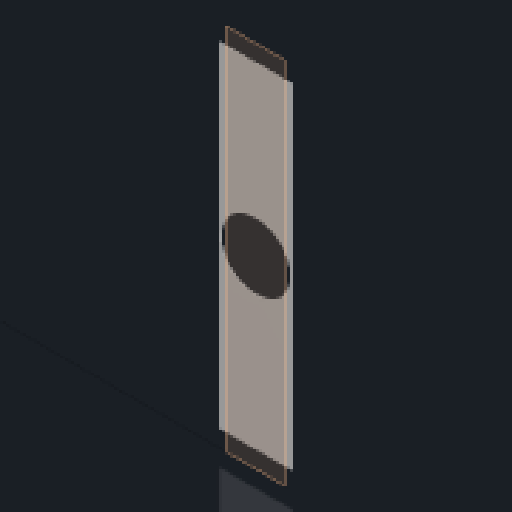
# Autodesk Inventor part: CARCASA_ALUM_2
Saved by Autodesk Inventor 2024.3 (Build 283343000, 343)
## iProperties
Created: 2024-05-15
Part Number: CARCASA_ALUM_2
Material: Generic
Document SubType Name: Sheet Metal
Designer: Niler
Density: 1 g/cm^3
Sheet Metal Rule: Default_mm
Appearance: Default
Author: Niler
Autodesk Inventor part; units mm, degrees
ref_plane "YZ Plane" through (0, 0, 0) normal (1, 0, 0) x (0, 1, 0)
ref_plane "XZ Plane" through (0, 0, 0) normal (0, 1, 0) x (-1, 0, 0)
ref_plane "XY Plane" through (0, 0, 0) normal (0, 0, 1) x (1, 0, 0)
ref_plane "Work Plane1" through (0, 0, 0) normal (0, 0, 1) x (1, 0, 0)
sketch "Sketch1" plane through (0, 0, 0) normal (0, 0, 1) x (1, 0, 0)
  line L0 (-90.0071, -785) -> (-90.0071, 235)
  line L1 (134.6291, -785) -> (-90.0071, -785)
  line L2 (134.6291, -785) -> (134.6291, 235)
  line L3 (-90.0071, 235) -> (134.6291, 235)
  spline S0 degree 3 poles (-83.4665, -275) (-83.4665, -270.5526) (-82.9168, -262.7698) (-81.2022, -254.0249) (-79.4626, -247.5768) (-78.0785, -243.3409) (-76.0752, -238.1427) (-74.2575, -234.0687) (-71.7257, -229.0988) (-69.4967, -225.2274) (-66.4671, -220.5344) (-63.8533, -216.9028) (-60.3609, -212.5309) (-57.3922, -209.1725) (-53.4761, -205.1609) (-50.1847, -202.1053) (-45.8867, -198.4886) (-42.3073, -195.7614) (-37.6715, -192.5693) (-33.84, -190.1925) (-28.9123, -187.4503) (-24.8659, -185.4423) (-19.6933, -183.1709) (-15.4701, -181.5469) (-10.1006, -179.7632) (-5.7393, -178.5349) (-0.2217, -177.2517) (4.2386, -176.428) (9.8552, -175.6545) (14.375, -175.2412) (20.0412, -174.9828) (24.5808, -174.9828) (30.247, -175.2412) (34.7668, -175.6545) (40.3834, -176.428) (44.8437, -177.2517) (50.3613, -178.5349) (54.7226, -179.7632) (60.092, -181.5469) (64.3153, -183.1709) (69.4878, -185.4423) (73.5343, -187.4503) (78.4619, -190.1925) (82.2935, -192.5693) (86.9292, -195.7614) (90.5087, -198.4886) (94.8067, -202.1053) (98.098, -205.1609) (102.0141, -209.1725) (104.9829, -212.5309) (108.4753, -216.9028) (111.089, -220.5344) (114.1187, -225.2274) (116.3477, -229.0988) (118.8794, -234.0687) (120.6972, -238.1427) (122.7004, -243.3409) (124.0846, -247.5768) (125.5343, -252.9502) (126.4672, -257.3042) (127.3447, -262.7966) (127.8142, -267.2225) (128.108, -272.775) (128.108, -277.225) (127.8142, -282.7775) (127.3447, -287.2034) (126.4672, -292.6958) (125.5343, -297.0498) (124.0846, -302.4232) (122.7004, -306.6591) (120.6972, -311.8573) (118.8794, -315.9313) (116.3477, -320.9012) (114.1187, -324.7726) (111.089, -329.4656) (108.4753, -333.0972) (104.9829, -337.4691) (102.0141, -340.8275) (98.098, -344.8391) (94.8067, -347.8947) (90.5087, -351.5114) (86.9292, -354.2386) (82.2935, -357.4307) (78.4619, -359.8075) (73.5343, -362.5497) (69.4878, -364.5577) (64.3153, -366.8291) (60.092, -368.4531) (54.7226, -370.2368) (50.3613, -371.4651) (44.8437, -372.7483) (40.3834, -373.572) (34.7668, -374.3455) (30.247, -374.7588) (24.5808, -375.0172) (20.0412, -375.0172) (14.375, -374.7588) (9.8552, -374.3455) (4.2386, -373.572) (-0.2217, -372.7483) (-5.7393, -371.4651) (-10.1006, -370.2368) (-15.4701, -368.4531) (-19.6933, -366.8291) (-24.8659, -364.5577) (-28.9123, -362.5497) (-33.84, -359.8075) (-37.6715, -357.4307) (-42.3073, -354.2386) (-45.8867, -351.5114) (-50.1847, -347.8947) (-53.4761, -344.8391) (-57.3922, -340.8275) (-60.3609, -337.4691) (-63.8533, -333.0972) (-66.4671, -329.4656) (-69.4967, -324.7726) (-71.7257, -320.9012) (-74.2575, -315.9313) (-76.0752, -311.8573) (-78.0785, -306.6591) (-79.4626, -302.4232) (-81.2022, -295.9751) (-82.9168, -287.2302) (-83.4665, -279.4474) (-83.4665, -275) knots -6.283185 -6.283185 -6.283185 -6.283185 -6.152286 -6.054111 -6.021386 -5.955936 -5.923211 -5.857761 -5.825036 -5.759587 -5.726862 -5.661412 -5.628687 -5.563237 -5.530512 -5.465062 -5.432337 -5.366887 -5.334163 -5.268713 -5.235988 -5.170538 -5.137813 -5.072363 -5.039638 -4.974188 -4.941463 -4.876014 -4.843289 -4.777839 -4.745114 -4.679664 -4.646939 -4.581489 -4.548764 -4.483315 -4.45059 -4.38514 -4.352415 -4.286965 -4.25424 -4.18879 -4.156065 -4.090615 -4.057891 -3.992441 -3.959716 -3.894266 -3.861541 -3.796091 -3.763366 -3.697916 -3.665191 -3.599742 -3.567017 -3.501567 -3.468842 -3.403392 -3.370667 -3.305217 -3.272492 -3.207043 -3.174318 -3.108868 -3.076143 -3.010693 -2.977968 -2.912518 -2.879793 -2.814343 -2.781618 -2.716169 -2.683444 -2.617994 -2.585269 -2.519819 -2.487094 -2.421644 -2.388919 -2.32347 -2.290745 -2.225295 -2.19257 -2.12712 -2.094395 -2.028945 -1.99622 -1.93077 -1.898046 -1.832596 -1.799871 -1.734421 -1.701696 -1.636246 -1.603521 -1.538071 -1.505346 -1.439897 -1.407172 -1.341722 -1.308997 -1.243547 -1.210822 -1.145372 -1.112647 -1.047198 -1.014473 -0.949023 -0.916298 -0.850848 -0.818123 -0.752673 -0.719948 -0.654498 -0.621774 -0.556324 -0.523599 -0.458149 -0.425424 -0.359974 -0.327249 -0.261799 -0.229074 -0.1309 0 0 0 0
  point P0 (0, 0)
  point P1 (-83.4665, -275)
extrude "Plate1" add sketch "Sketch1" against normal blind 1.5
equation "\"d0\" = Thickness"
equation "\"BendRadius\" = Thickness"
equation "\"BendReliefWidth\" = Thickness"
equation "\"BendReliefDepth\" = 0.5 * Thickness"
equation "\"CornerReliefSize\" = 4 * Thickness"
equation "\"MinimumRemnant\" = 2 * Thickness"
equation "\"TransitionRadius\" = BendRadius"
equation "\"JacobiRadiusSize\" = BendRadius"
equation "\"GapSize\" = Thickness"
equation "\"Thickness\" = 1.5"
body "Solid1"
